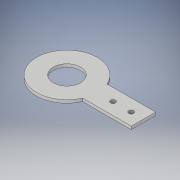
# Autodesk Inventor part: wheel tip
Saved by Autodesk Inventor 2019 (Build 230136000, 136)
## iProperties
Created: 2019-01-18
Part Number: wheel tip
Material: Generic
Document SubType Name: Modeling
Designer: s-2513225
Density: 1 g/cm^3
Appearance: Default
Author: s-2513225
Autodesk Inventor part; units mm, degrees
ref_plane "YZ Plane" through (0, 0, 0) normal (1, 0, 0) x (0, 1, 0)
ref_plane "XZ Plane" through (0, 0, 0) normal (0, 1, 0) x (-1, 0, 0)
ref_plane "XY Plane" through (0, 0, 0) normal (0, 0, 1) x (1, 0, 0)
sketch "Sketch1" plane through (0, 0, 0) normal (0, 1, 0) x (-1, 0, 0)
  line L0 (0, 0) -> (0, -12.7)
  line L1 (0, -12.7) -> (50.8, -12.7)
  line L2 (0, 0) -> (0, 12.7)
  line L3 (0, 12.7) -> (50.8, 12.7)
  line L4 (54.4994, 0) -> (79.8994, 0) construction
  arc A0 (50.8, -12.7) -> (50.8, 12.7) centre (79.8994, 0) ccw
  line L5 (0, 0) -> (12.7, 0) construction
  line L6 (12.7, 0) -> (31.75, 0) construction
  circle A1 centre (12.7, 0) radius 2.5797
  circle A2 centre (31.75, 0) radius 2.5797
  circle A3 centre (79.8994, 0) radius 14.2875
  dimension "d0" = 12.7
  dimension "d1" = 50.8
  dimension "d5" = 12.7
  dimension "d6" = 19.05
  dimension "d7" = 5.1594
  dimension "d8" = 5.1594
  dimension "d9" = 28.575
  dimension "d12" = 12.7
  constraints: 14 end point, 4 centre point, 4 coincident, 2 horizontal, 2 point on circle, 1 perpendicular, 1 point on line, 1 vertical
  measures "d0" distance of L0.start L0.end
  measures "d1" distance of L0.end L1.end
  measures "d5" distance of L0.start L5.end
  measures "d6" distance of L5.end L6.end
  measures "d7" diameter of A1
  measures "d8" diameter of A2
  measures "d9" diameter of A3
  measures "d12" distance of L0.start L3.start
extrude "Extrusion1" add sketch "Sketch1" along normal blind 3.175
body "Solid1"
